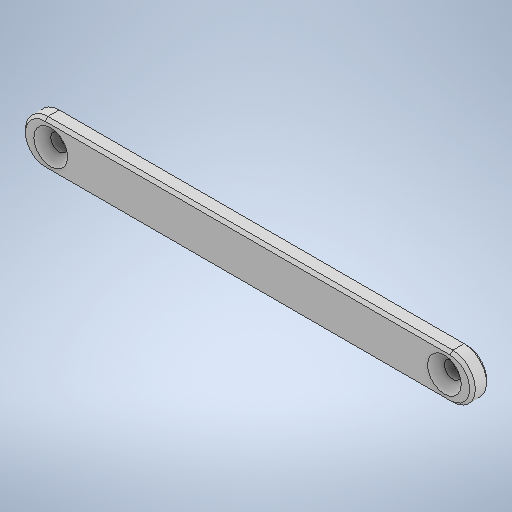
# Autodesk Inventor part: HoldingPlate
Saved by Autodesk Inventor 2025.2 (Build 292293000, 293)
## iProperties
Created: 2025-08-15
Part Number: HoldingPlate
Material: Generic
Document SubType Name: Modeling
Designer: hofma
Density: 1 g/cm^3
Appearance: Default
Author: hofma
Autodesk Inventor part; units mm, degrees
ref_plane "YZ Plane" through (0, 0, 0) normal (1, 0, 0) x (0, 1, 0)
ref_plane "XZ Plane" through (0, 0, 0) normal (0, 1, 0) x (-1, 0, 0)
ref_plane "XY Plane" through (0, 0, 0) normal (0, 0, 1) x (1, 0, 0)
sketch "Sketch1" plane through (0, 0, 0) normal (0, 0, 1) x (1, 0, 0)
  line L0 (-40, 4) -> (40, 4)
  line L1 (40, 4) -> (40, -4)
  line L2 (40, -4) -> (-40, -4)
  line L3 (-40, -4) -> (-40, 4)
  line L4 (-40, 4) -> (40, -4) construction
  line L5 (40, 4) -> (-40, -4) construction
  line L6 (0, 0) -> (0, 15.184) construction
  circle A0 centre (-35, 0) radius 1.5
  circle A1 centre (35, 0) radius 1.5
  dimension "d0" = 3
  dimension "d1" = 70
  dimension "d2" = 80
  dimension "d3" = 8
  constraints: 14 end point, 2 centre point, 2 midpoint, 2 parallel, 1 horizontal, 1 horizontal alignment, 1 perpendicular, 1 vertical, 1 other
  measures "d0" diameter of A0
  measures "d1" distance of A1.centre A0.centre
  measures "d2" distance between parallel lines of L1 L3
  measures "d3" distance between parallel lines of L2 L0
extrude "Extrusion1" add sketch "Sketch1" along normal blind 3
chamfer "Chamfer1" distance 1.5 angle 45 2 edges at (-36.5, 0, 3) (33.5, 0, 3)
fillet "Fillet1" radius 4 4 edges at (-40, 4, 1.5) (-40, -4, 1.5) (40, 4, 1.5) (40, -4, 1.5)
chamfer "Chamfer2" distance 0.5 angle 45 8 edges at (0, 4, 0) (-38.8286, 2.8286, 0) (0, -4, 0) (38.8286, 2.8286, 0) (0, 4, 3) (-38.8286, 2.8286, 3) (0, -4, 3) (38.8286, 2.8286, 3)
body "Solid1"
